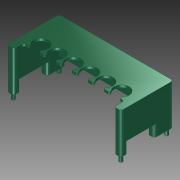
# Autodesk Inventor part: DispProtecc
Saved by Autodesk Inventor 2015 (Build 190159000, 159)
## iProperties
Created: 2018-05-08
Part Number: DispProtecc
Material: PC/ABS Plastic
Document SubType Name: Modeling
Designer: Silas
Density: 0.357273 g/cm^3
Appearance: Smooth - Dark Sea Green
Author: Silas
Autodesk Inventor part; units mm, degrees
ref_plane "YZ Plane" through (0, 0, 0) normal (1, 0, 0) x (0, 1, 0)
ref_plane "XZ Plane" through (0, 0, 0) normal (0, 1, 0) x (-1, 0, 0)
ref_plane "XY Plane" through (0, 0, 0) normal (0, 0, 1) x (1, 0, 0)
sketch "Sketch1" plane through (0, 0, 0) normal (0, 0, 1) x (1, 0, 0)
  line L0 (-49.53, 22.7012) -> (49.53, 22.7013)
  line L1 (49.53, 22.7013) -> (49.53, -22.7012)
  line L2 (49.53, -22.7012) -> (-49.53, -22.7013)
  line L3 (-49.53, -22.7013) -> (-49.53, 22.7012)
  line L4 (0, 22.7013) -> (0, -22.7013) construction
  line L5 (-49.53, 0) -> (49.53, 0) construction
  line L6 (-49.53, -7.5375) -> (49.53, -7.5375) construction
  circle A0 centre (-34.925, -7.5375) radius 6.5
  circle A1 centre (-20.955, -7.5375) radius 6.5
  circle A2 centre (-6.985, -7.5375) radius 6.5
  circle A3 centre (6.985, -7.5375) radius 6.5
  circle A4 centre (20.955, -7.5375) radius 6.5
  circle A5 centre (34.925, -7.5375) radius 6.5
  point P0 (0, 0)
  dimension "d0" = 99.06
  dimension "d1" = 45.4025
  dimension "d2" = 15.1638
  dimension "d3" = 13
  dimension "d4" = 13
  dimension "d5" = 13
  dimension "d6" = 13
  dimension "d7" = 13
  dimension "d8" = 13
  dimension "d9" = 14.605
  dimension "d10" = 28.575
  dimension "d11" = 42.545
  dimension "d12" = 56.515
  dimension "d13" = 70.485
  dimension "d14" = 84.455
  constraints: 14 end point, 8 point on line, 6 centre point, 6 midpoint, 2 parallel, 2 perpendicular, 1 horizontal
  measures "d0" distance of L1.end L2.end
  measures "d1" distance of L0.end L1.end
  measures "d2" distance between parallel lines of L2 L6
  measures "d3" diameter of A0
  measures "d4" diameter of A1
  measures "d5" diameter of A2
  measures "d6" diameter of A3
  measures "d7" diameter of A4
  measures "d8" diameter of A5
  measures "d9" distance from line of L3 A0.centre
  measures "d10" distance from line of L3 A1.centre
  measures "d11" distance from line of L3 A2.centre
  measures "d12" distance from line of L3 A3.centre
  measures "d13" distance from line of L3 A4.centre
  measures "d14" distance from line of L3 A5.centre
extrude "Extrusion1" add sketch "Sketch1" along normal blind 2
fillet "Fillet1" radius 2.286 4 edges at (49.53, 22.7013, 1) (49.53, -22.7012, 1) (-49.53, -22.7013, 1) (-49.53, 22.7012, 1)
sketch "Sketch2" plane through (0, 0, 0) normal (0, 0, -1) x (-1, 0, 0)
  arc A0 (49.53, 20.4152) -> (47.244, 22.7012) centre (47.244, 20.4152) ccw projected
  line L0 (47.244, 22.7012) -> (-47.244, 22.7013) projected
  arc A1 (-47.244, 22.7013) -> (-49.53, 20.4153) centre (-47.244, 20.4153) ccw projected
  line L1 (-49.53, 20.4153) -> (-49.53, -20.4152) projected
  arc A2 (-49.53, -20.4152) -> (-47.244, -22.7012) centre (-47.244, -20.4153) ccw projected
  line L2 (-47.244, -22.7012) -> (47.244, -22.7013) projected
  arc A3 (47.244, -22.7013) -> (49.53, -20.4153) centre (47.244, -20.4153) ccw projected
  line L3 (49.53, -20.4153) -> (49.53, 20.4152) projected
  circle A4 centre (-34.925, -7.5375) radius 6.5 projected
  circle A5 centre (-20.955, -7.5375) radius 6.5 projected
  circle A6 centre (-6.985, -7.5375) radius 6.5 projected
  circle A7 centre (6.985, -7.5375) radius 6.5 projected
  circle A8 centre (20.955, -7.5375) radius 6.5 projected
  circle A9 centre (34.925, -7.5375) radius 6.5 projected
  arc A10 (47.625, 20.4152) -> (47.244, 20.7962) centre (47.244, 20.4152) ccw
  line L4 (47.244, 20.7962) -> (-47.244, 20.7963)
  arc A11 (-47.244, 20.7963) -> (-47.625, 20.4152) centre (-47.244, 20.4153) ccw
  line L5 (-47.625, 20.4152) -> (-47.625, -20.4152)
  arc A12 (-47.625, -20.4152) -> (-47.244, -20.7962) centre (-47.244, -20.4153) ccw
  line L6 (-47.244, -20.7962) -> (47.244, -20.7963)
  arc A13 (47.244, -20.7963) -> (47.625, -20.4152) centre (47.244, -20.4153) ccw
  line L7 (47.625, -20.4152) -> (47.625, 20.4152)
  line L8 (43.53, 16.7012) -> (-43.53, 16.7013)
  line L9 (-43.53, 16.7013) -> (-43.53, -16.7013)
  line L10 (-43.53, -16.7013) -> (43.53, -16.7013)
  line L11 (43.53, -16.7013) -> (43.53, 16.7012)
  point P0 (0, 0)
  dimension "d18" = 1.905
  dimension "d26" = 6
  constraints: 16 end point, 8 point on circle, 4 centre point, 10 other
  measures "d18" distance between parallel lines of L3 L7
  measures "d26" distance between parallel lines of L3 L11
extrude "Extrusion2" add sketch "Sketch2" along normal blind 33 contours L3 A3 L2 A2 L1 A1 L0 A0 | L7 A13 L6 A12 L5 A11 L4 A10
sketch "Sketch3" plane through (0, 0, 2) normal (0, 0, 1) x (1, 0, 0)
  circle A0 centre (34.925, -7.5375) radius 6.5 projected
  circle A1 centre (20.955, -7.5375) radius 6.5 projected
  circle A2 centre (6.985, -7.5375) radius 6.5 projected
  circle A3 centre (-6.985, -7.5375) radius 6.5 projected
  circle A4 centre (-20.955, -7.5375) radius 6.5 projected
  circle A5 centre (-34.925, -7.5375) radius 6.5 projected
  arc A6 (-47.244, 22.7012) -> (-49.53, 20.4152) centre (-47.244, 20.4152) ccw projected
  line L0 (-49.53, 20.4152) -> (-49.53, -20.4153) projected
  arc A7 (-49.53, -20.4153) -> (-47.244, -22.7013) centre (-47.244, -20.4153) ccw projected
  line L1 (-47.244, -22.7013) -> (47.244, -22.7012) projected
  arc A8 (47.244, -22.7012) -> (49.53, -20.4152) centre (47.244, -20.4153) ccw projected
  line L2 (49.53, -20.4152) -> (49.53, 20.4153) projected
  arc A9 (49.53, 20.4153) -> (47.244, 22.7013) centre (47.244, 20.4153) ccw projected
  line L3 (47.244, 22.7013) -> (-47.244, 22.7012) projected
  line L4 (-43.53, -22.7013) -> (43.53, -22.7013)
  line L5 (43.53, -22.7013) -> (43.53, -13.7013)
  line L6 (43.53, -13.7013) -> (-43.53, -13.7013)
  line L7 (-43.53, -13.7013) -> (-43.53, -22.7013)
  line L8 (-47.244, -22.7013) -> (47.244, -22.7012) projected
  line L9 (43.53, 16.7013) -> (43.53, -16.7013) projected
  line L10 (43.53, -16.7013) -> (-43.53, -16.7013) projected
  line L11 (-43.53, -16.7013) -> (-43.53, 16.7012) projected
  point P0 (0, 0)
  point P1 (0, -22.7013)
  point P2 (0, -22.7013)
  point P3 (-43.53, -18.2013)
  point P4 (43.53, -18.2013)
  dimension "d21" = 9
  constraints: 8 end point, 6 midpoint, 2 parallel, 2 point on line, 1 horizontal, 1 perpendicular
  measures "d21" distance between parallel lines of L1 L6
extrude "Extrusion3" cut sketch "Sketch3" against normal through all contours L6 A0 | A0 L6 L5 L10 L7 A5 A4 A3 A2 A1 | A1 L6 | L5 L1 L7 L10 | A2 L6 | A3 L6 | L6 A5 | A4 L6 picked at (34.6921, -13.8008) picked at (21.1879, -13.8008) picked at (6.7521, -13.8008) picked at (-6.7521, -13.8008) picked at (-35.1579, -13.8008) picked at (-20.7221, -13.8008)
fillet "Fillet2" radius 1 12 edges at (-32.8616, -13.7013, 1) (-36.9884, -13.7013, 1) (-18.8916, -13.7013, 1) (-23.0184, -13.7013, 1) (-4.9216, -13.7013, 1) (-9.0484, -13.7013, 1) (9.0484, -13.7013, 1) (4.9216, -13.7013, 1) (23.0184, -13.7013, 1) (18.8916, -13.7013, 1) (36.9884, -13.7013, 1) (32.8616, -13.7013, 1)
sketch "Sketch4" plane through (0, 0, -33) normal (0, 0, -1) x (-1, 0, 0)
  line L0 (43.53, 16.7012) -> (43.53, -22.7013) projected
  arc A0 (47.244, -22.7013) -> (49.53, -20.4153) centre (47.244, -20.4153) ccw projected
  line L1 (49.53, -20.4153) -> (49.53, 20.4152) projected
  arc A1 (49.53, 20.4152) -> (47.244, 22.7012) centre (47.244, 20.4152) ccw projected
  line L2 (47.244, 22.7012) -> (-47.244, 22.7013) projected
  arc A2 (-47.244, 22.7013) -> (-49.53, 20.4153) centre (-47.244, 20.4153) ccw projected
  line L3 (-49.53, 20.4153) -> (-49.53, -20.4152) projected
  arc A3 (-49.53, -20.4152) -> (-47.244, -22.7012) centre (-47.244, -20.4153) ccw projected
  line L4 (-43.53, -22.7013) -> (-43.53, 16.7013) projected
  circle A4 centre (-46.6725, 19.8438) radius 1.485
  line L5 (-43.53, 16.7013) -> (43.53, 16.7012) projected
  line L6 (43.53, -22.7013) -> (47.244, -22.7013) projected
  line L7 (-47.244, -22.7012) -> (-43.53, -22.7013) projected
  circle A5 centre (-46.6725, -19.8438) radius 1.485
  circle A6 centre (46.6725, -19.8438) radius 1.485
  circle A7 centre (46.6725, 19.8437) radius 1.485
  point P0 (0, 0)
  dimension "d25" = 2.97
  dimension "d27" = 2.8575
  dimension "d28" = 2.8575
  dimension "d29" = 2.97
  dimension "d30" = 2.97
  dimension "d31" = 2.97
  dimension "d32" = 2.8575
  dimension "d33" = 2.8575
  dimension "d34" = 2.8575
  dimension "d35" = 2.8575
  dimension "d36" = 2.8575
  dimension "d37" = 2.8575
  constraints: 4 centre point
  measures "d25" diameter of A4
  measures "d27" distance from line of A4.centre L3
  measures "d28" distance from line of A4.centre L2
  measures "d29" diameter of A5
  measures "d30" diameter of A6
  measures "d31" diameter of A7
  measures "d32" distance from line of A7.centre L2
  measures "d33" distance from line of A7.centre L1
  measures "d34" distance from line of A5.centre L3
  measures "d35" distance from line of A6.centre L1
  measures "d36" distance from line of A6.centre L6
  measures "d37" distance from line of A5.centre L7
extrude "Extrusion4" add sketch "Sketch4" along normal blind 6 contours A4 | A5 | A6 | A7
fillet "Fillet3" radius 2.286 4 edges at (-43.53, -22.7013, -15.5) (-43.53, -13.7013, 1) (43.53, -13.7013, 1) (43.53, -22.7013, -15.5)
sketch "Sketch5" plane through (0, 0, -33) normal (0, 0, -1) x (-1, 0, 0)
  circle A0 centre (46.6725, 19.8437) radius 1.485 projected
  circle A1 centre (-46.6725, -19.8438) radius 1.485 projected
  circle A2 centre (-46.6725, 19.8438) radius 1.485 projected
  circle A3 centre (46.6725, -19.8438) radius 1.485 projected
  arc A4 (-45.816, -22.7012) -> (-43.53, -20.4153) centre (-45.816, -20.4153) ccw projected
  line L0 (-43.53, -20.4153) -> (-43.53, 16.7013) projected
  line L1 (-43.53, 16.7013) -> (43.53, 16.7012) projected
  line L2 (43.53, 16.7012) -> (43.53, -20.4153) projected
  arc A5 (43.53, -20.4153) -> (45.816, -22.7013) centre (45.816, -20.4153) ccw projected
  line L3 (45.816, -22.7013) -> (47.244, -22.7013) projected
  arc A6 (47.244, -22.7013) -> (49.53, -20.4153) centre (47.244, -20.4153) ccw projected
  line L4 (49.53, -20.4153) -> (49.53, 20.4152) projected
  arc A7 (49.53, 20.4152) -> (47.244, 22.7012) centre (47.244, 20.4152) ccw projected
  line L5 (47.244, 22.7012) -> (-47.244, 22.7013) projected
  arc A8 (-47.244, 22.7013) -> (-49.53, 20.4153) centre (-47.244, 20.4153) ccw projected
  line L6 (-49.53, 20.4153) -> (-49.53, -20.4152) projected
  arc A9 (-49.53, -20.4152) -> (-47.244, -22.7012) centre (-47.244, -20.4153) ccw projected
  line L7 (-47.244, -22.7012) -> (-45.816, -22.7012) projected
  line L8 (-49.53, -20.4152) -> (-49.53, 20.4153) projected
  line L9 (-43.53, -20.4153) -> (-43.53, 16.7013) projected
  line L10 (-49.53, -16.7012) -> (-43.53, -16.7012)
  line L11 (-43.53, -16.7012) -> (-43.53, 6.2988)
  line L12 (-43.53, 6.2988) -> (-49.53, 6.2988)
  line L13 (-49.53, 6.2988) -> (-49.53, -16.7012)
  line L14 (49.53, -20.4153) -> (49.53, 20.4152) projected
  line L15 (43.53, -15.9873) -> (43.53, 16.7012) projected
  line L16 (49.53, -16.7013) -> (43.53, -16.7013)
  line L17 (43.53, -16.7013) -> (43.53, 6.2987)
  line L18 (43.53, 6.2987) -> (49.53, 6.2987)
  line L19 (49.53, 6.2987) -> (49.53, -16.7013)
  line L20 (43.53, 16.7012) -> (-43.53, 16.7013) projected
  line L21 (-47.244, 22.7013) -> (47.244, 22.7012) projected
  line L22 (43.53, 16.7012) -> (-43.53, 16.7013)
  line L23 (-43.53, 16.7013) -> (-43.53, 22.7013)
  line L24 (-43.53, 22.7013) -> (43.53, 22.7013)
  line L25 (43.53, 22.7013) -> (43.53, 16.7012)
  point P0 (0, 0)
  dimension "d41" = 23
  dimension "d42" = 6
  dimension "d43" = 6
  dimension "d44" = 23
  dimension "d45" = 0
  dimension "d46" = 0
  constraints: 24 end point, 6 parallel, 6 point on line, 3 horizontal, 3 perpendicular
  measures "d41" distance between parallel lines of L12 L10
  measures "d42" distance between parallel lines of L7 L10
  measures "d43" distance between parallel lines of L3 L16
  measures "d44" distance between parallel lines of L16 L18
  measures "d45" distance between parallel lines of L0 L23
  measures "d46" distance between parallel lines of L25 L15
extrude "Extrusion5" cut sketch "Sketch5" against normal blind 10 contours L10 L6 L12 L0 | L23 L5 L25 L1 | L18 L4 L16 L2
fillet "Fillet4" radius 2.286 10 edges at (-43.53, -16.7013, -28) (-49.53, -16.7013, -28) (-49.53, 6.2987, -28) (-43.53, 6.2987, -28) (49.53, -16.7012, -28) (43.53, -16.7012, -28) (49.53, 6.2988, -28) (43.53, 6.2988, -28) (-43.53, 22.7013, -28) (43.53, 22.7013, -28)
chamfer "Chamfer1" distance 0.5 angle 45 4 edges at (-45.1875, -19.8438, -39) (48.1575, -19.8438, -39) (48.1575, 19.8438, -39) (-45.1875, 19.8437, -39)
sketch "Sketch7" plane through (-46.6725, -19.8438, -39) normal (0, 0, -1) x (-1, 0, 0)
  circle A0 centre (0, 0) radius 1.485 projected
  circle A1 centre (0, 39.6875) radius 1.485 projected
  circle A2 centre (-93.345, 39.6875) radius 1.485 projected
  circle A3 centre (-93.345, 0) radius 1.485 projected
  point P0 (-46.6725, 19.8438)
extrude "Extrusion6" [suppressed]
equation "\"d28\" = d27"
equation "\"d29\" = d25"
equation "\"d30\" = d25"
equation "\"d31\" = d25"
equation "\"d32\" = d28"
equation "\"d33\" = d32"
equation "\"d34\" = d27"
equation "\"d35\" = d34"
equation "\"d36\" = d35"
equation "\"d37\" = d34"
equation "\"d43\" = d42"
equation "\"d44\" = d41"
body "Solid1"
